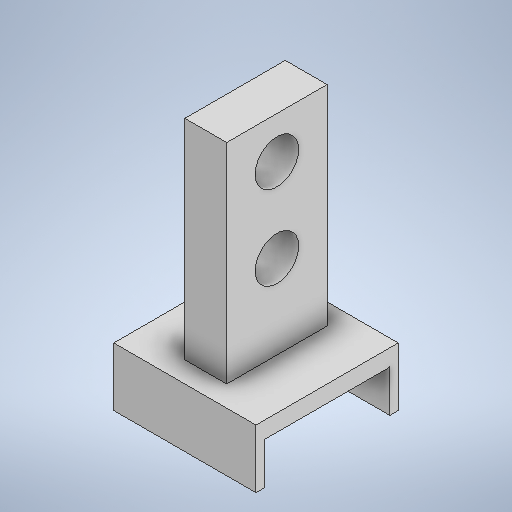
# Autodesk Inventor part: 差分線圈上蓋
Saved by Autodesk Inventor 2025.2 (Build 292293000, 293)
## iProperties
Created: 2025-07-16
Part Number: 差分線圈上蓋
Material: 一般
Document SubType Name: Modeling
Designer: 123
Density: 1 g/cm^3
Appearance: 預設
Author: 123
Autodesk Inventor part; units mm, degrees
ref_plane "YZ Plane" through (0, 0, 0) normal (1, 0, 0) x (0, 1, 0)
ref_plane "XZ Plane" through (0, 0, 0) normal (0, 1, 0) x (-1, 0, 0)
ref_plane "XY Plane" through (0, 0, 0) normal (0, 0, 1) x (1, 0, 0)
sketch "草圖1" plane through (0, 0, 0) normal (0, 1, 0) x (-1, 0, 0)
  line L0 (8.5, 8.5) -> (-8.5, 8.5)
  line L1 (-8.5, 8.5) -> (-8.5, -8.5)
  line L2 (-8.5, -8.5) -> (8.5, -8.5)
  line L3 (8.5, -8.5) -> (8.5, 8.5)
  line L4 (8.5, 8.5) -> (-8.5, -8.5) construction
  line L5 (-8.5, 8.5) -> (8.5, -8.5) construction
  point P0 (0, 0)
  dimension "d0" = 17
  dimension "d1" = 17
  constraints: 12 end point, 2 midpoint, 2 parallel, 1 horizontal, 1 perpendicular
  measures "d0" distance of L2.end L0.start
  measures "d1" distance of L0.start L0.end
extrude "擠出1" add sketch "草圖1" along normal blind 2
sketch "草圖3" plane through (0, 0, 0) normal (0, -1, 0) x (1, 0, 0)
  line L0 (-4.4, 2.5) -> (-2.5, 2.5)
  line L1 (-2.5, 2.5) -> (-2.5, -2.5)
  line L2 (-2.5, -2.5) -> (-4.4, -2.5)
  line L3 (-4.4, -2.5) -> (-4.4, 2.5)
  line L4 (-4.4, 2.5) -> (-2.5, -2.5) construction
  line L5 (-2.5, 2.5) -> (-4.4, -2.5) construction
  line L6 (2.5, 2.5) -> (4.4, 2.5)
  line L7 (4.4, 2.5) -> (4.4, -2.5)
  line L8 (4.4, -2.5) -> (2.5, -2.5)
  line L9 (2.5, -2.5) -> (2.5, 2.5)
  line L10 (2.5, 2.5) -> (4.4, -2.5) construction
  line L11 (4.4, 2.5) -> (2.5, -2.5) construction
  point P0 (0, 0)
  point P1 (-3.45, 0)
  point P2 (3.45, 0)
  dimension "d4" = 1.9
  dimension "d5" = 1.9
  dimension "d6" = 5
  dimension "d7" = 5
  dimension "d8" = 0
  dimension "d9" = 5
  dimension "d10" = 2.5
  constraints: 24 end point, 4 midpoint, 4 parallel, 2 horizontal, 2 perpendicular, 1 point on line
  measures "d4" distance of L0.start L0.end
  measures "d5" distance of L6.start L6.end
  measures "d6" distance of L6.end L7.end
  measures "d7" distance of L2.end L0.start
  measures "d8" vertical distance of point (0, 0) point (-3.45, 0)
  measures "d9" distance between parallel lines of L9 L1
  measures "d10" distance from line of point (0, 0) L1
extrude "擠出2" add sketch "草圖3" along normal blind 1
sketch "草圖4" plane through (0, 0, 0) normal (0, -1, 0) x (1, 0, 0)
  line L0 (-8.5, -8.5) -> (-8.5, 8.5) projected
  line L1 (8.5, 8.5) -> (8.5, -8.5) projected
  line L2 (-8.5, 8.5) -> (8.5, 8.5)
  line L3 (8.5, 8.5) -> (8.5, 7.5)
  line L4 (8.5, 7.5) -> (-8.5, 7.5)
  line L5 (-8.5, 7.5) -> (-8.5, 8.5)
  line L6 (-8.5, -7.5) -> (8.5, -7.5)
  line L7 (8.5, -7.5) -> (8.5, -8.5)
  line L8 (8.5, -8.5) -> (-8.5, -8.5)
  line L9 (-8.5, -8.5) -> (-8.5, -7.5)
  point P0 (0, 0)
  point P1 (-8.5, -7.5)
  point P2 (-8.5, 7.5)
  dimension "d13" = 1
  dimension "d14" = 1
  constraints: 16 end point, 4 parallel, 2 horizontal, 2 perpendicular, 2 point on line
  measures "d13" distance between parallel lines of L4 L2
  measures "d14" distance between parallel lines of L8 L6
extrude "擠出3" add sketch "草圖4" along normal blind 5 contours L0 L6 L1 L8 | L0 L2 L1 L4
sketch "草圖5" plane through (8.5, 0, 7.5) normal (0, 0, -1) x (-1, 0, 0)
  line L0 (10.5, -12) -> (6.5, -12)
  line L1 (6.5, -12) -> (6.5, 2)
  line L2 (6.5, 2) -> (10.5, 2)
  line L3 (10.5, 2) -> (10.5, -12)
  line L4 (0, -5) -> (17, -5) projected
  line L5 (10.5, -12) -> (6.5, 2) construction
  line L6 (6.5, -12) -> (10.5, 2) construction
  point P0 (8.5, 0)
  point P1 (8.5, -5)
  point P2 (6.5, -5)
  point P3 (10.5, -5)
  dimension "d17" = 14
  dimension "d18" = 4
  constraints: 12 end point, 3 midpoint, 2 parallel, 1 horizontal, 1 perpendicular
  measures "d17" distance of L2.end L0.start
  measures "d18" distance of L1.end L2.end
extrude "擠出4" add sketch "草圖5" along normal blind 1.5 contours L4 L1 L2 L3
sketch "草圖6" plane through (-8.5, 0, -7.5) normal (0, 0, 1) x (1, 0, 0)
  line L0 (6.5, 2) -> (10.5, 2)
  line L1 (10.5, 2) -> (10.5, -12)
  line L2 (10.5, -12) -> (6.5, -12)
  line L3 (6.5, -12) -> (6.5, 2)
  line L4 (10.5, -5) -> (6.5, -5) projected
  line L5 (6.5, 2) -> (10.5, -12) construction
  line L6 (10.5, 2) -> (6.5, -12) construction
  point P0 (8.5, 0)
  point P1 (8.5, -5)
  point P2 (10.5, -7)
  point P3 (6.5, -7)
  dimension "d21" = 14
  dimension "d22" = 4
  constraints: 12 end point, 3 midpoint, 2 parallel, 1 horizontal, 1 perpendicular
  measures "d21" distance of L0.end L1.end
  measures "d22" distance of L1.end L2.end
extrude "擠出5" add sketch "草圖6" along normal blind 1.5 contours L0 L1 L4 L3
sketch "草圖7" plane through (0, 2, 0) normal (0, 1, 0) x (1, 0, 0)
  line L0 (-2.5, 6) -> (2.5, 6)
  line L1 (2.5, 6) -> (2.5, -6)
  line L2 (2.5, -6) -> (-2.5, -6)
  line L3 (-2.5, -6) -> (-2.5, 6)
  line L4 (-2.5, 6) -> (2.5, -6) construction
  line L5 (2.5, 6) -> (-2.5, -6) construction
  point P0 (0, 0)
  dimension "d25" = 12
  dimension "d26" = 5
  constraints: 12 end point, 2 midpoint, 2 parallel, 1 horizontal, 1 perpendicular
  measures "d25" distance of L0.end L1.end
  measures "d26" distance of L0.start L0.end
extrude "擠出6" add sketch "草圖7" along normal blind 25
sketch "草圖8" plane through (-2.5, 2, -6) normal (-1, 0, 0) x (0, 0, 1)
  circle A0 centre (6, 20) radius 2.6
  circle A1 centre (6, 10) radius 2.6
  line L0 (-2.5, 0) -> (14.5, 0) projected
  point P0 (6, -2)
  point P1 (6, 0)
  dimension "d29" = 5.2
  dimension "d30" = 5.2
  dimension "d31" = 10
  dimension "d32" = 10
  constraints: 2 centre point, 1 midpoint
  measures "d29" diameter of A0
  measures "d30" diameter of A1
  measures "d31" distance of point (6, 0) A1.centre
  measures "d32" distance of A1.centre A0.centre
extrude "擠出7" cut sketch "草圖8" against normal blind 25
